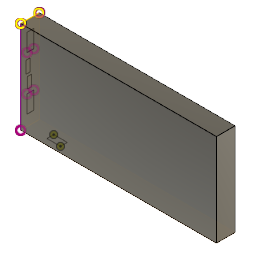
powerbank v11 (Autodesk Fusion 360 design; units mm, degrees)
Autodesk Fusion 360 part; units mm, degrees
box "BoxPrimitive1" add length 68.5 width 145 height 14 placed x (0, 0, -1) y (-1, 0, 0) z (0, 1, 0) at (145, 0, 0)
sketch "USB1" plane through (0, 0, 0) normal (-1, 0, 0) x (0, -1, 0)
  line L0 (-14, -68.5) -> (0, -68.5)
  line L1 (0, -68.5) -> (0, 0)
  line L2 (0, 0) -> (-14, 0)
  line L3 (-14, 0) -> (-14, -68.5)
  line L4 (-4.75, -60.5) -> (-9.75, -60.5)
  line L5 (-9.75, -60.5) -> (-9.75, -47.5)
  line L6 (-9.75, -47.5) -> (-4.75, -47.5)
  line L7 (-4.75, -47.5) -> (-4.75, -60.5)
  dimension "d14" = 5
  dimension "d15" = 13
  dimension "d16" = 8
  dimension "d17" = 4.25
  measures "d16" distance of L0 L4
  measures "d17" distance of L3 L5
extrude "Extrude USB1" cut sketch "USB1" against normal blind 20 contours L4 L5 L6 L7
sketch "USB4" plane through (0, 0, 0) normal (-1, 0, 0) x (0, -1, 0)
  line L0 (-14, -68.5) -> (0, -68.5)
  line L1 (0, -68.5) -> (0, 0)
  line L2 (-14, 0) -> (-14, -68.5)
  line L3 (-9.75, -21) -> (-4.75, -21)
  line L4 (-4.75, -21) -> (-4.75, -8)
  line L5 (-4.75, -8) -> (-9.75, -8)
  line L6 (-9.75, -8) -> (-9.75, -21)
  line L7 (0, 0) -> (-14, 0)
  dimension "d21" = 13
  dimension "d22" = 4.25
  dimension "d23" = 5
  dimension "d53" = 8
  measures "d21" distance of L3 L5
  measures "d22" distance of L2 L6
  measures "d23" distance of L4 L6
  measures "d53" distance of L5 L7
extrude "Extrude USB4" cut sketch "USB4" against normal blind 20 contours L3 L4 L5 L6
sketch "Sketch9" plane through (0, 0, 0) normal (-1, 0, 0) x (0, -1, 0)
  line L0 (-5, -44.5) -> (-8, -44.5)
  line L1 (-8, -44.5) -> (-8, -36.5)
  line L2 (-8, -36.5) -> (-5, -36.5)
  line L3 (-5, -36.5) -> (-5, -44.5)
  line L4 (0, -68.5) -> (0, 0)
  line L5 (-9.75, -47.5) -> (-4.75, -47.5)
  dimension "d34" = 8
  dimension "d35" = 3
  dimension "d36" = 5
  dimension "d37" = 3
  measures "d36" distance of L3 L4
  measures "d37" distance of L0 L5
extrude "Extrude4" cut sketch "Sketch9" against normal blind 10
sketch "Sketch10" plane through (0, 0, 0) normal (-1, 0, 0) x (0, -1, 0)
  line L0 (-4, -34.5) -> (-7, -34.5)
  line L1 (-7, -34.5) -> (-7, -25.5)
  line L2 (-7, -25.5) -> (-4, -25.5)
  line L3 (-4, -25.5) -> (-4, -34.5)
  line L4 (0, -68.5) -> (0, 0)
  line L5 (-9.75, -21) -> (-4.75, -21)
  dimension "d40" = 3
  dimension "d41" = 9
  dimension "d42" = 4
  dimension "d43" = 4.5
  measures "d42" distance of L3 L4
  measures "d43" distance of L2 L5
extrude "Extrude5" cut sketch "Sketch10" against normal blind 10
sketch "Sketch12" plane through (0, 0, 0) normal (0, 0, 1) x (-1, 0, 0)
  line L0 (0, 0) -> (-145, 0)
  line L1 (-145, 0) -> (-145, -14)
  line L2 (-145, -14) -> (0, -14)
  line L3 (0, 0) -> (0, -13.5)
sketch "Sketch15" plane through (0, 0, -68.5) normal (0, 0, -1) x (1, 0, 0)
  line L0 (145, -14) -> (145, 0)
  line L1 (145, 0) -> (0, 0)
  line L2 (0, 0) -> (0, -14)
  line L3 (0, -14) -> (145, -14)
  line L4 (15, -9.5) -> (25, -9.5)
  line L5 (25, -9.5) -> (25, -4.5)
  line L6 (25, -4.5) -> (15, -4.5)
  line L7 (15, -4.5) -> (15, -9.5)
